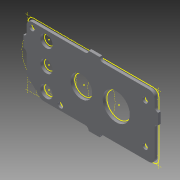
# Autodesk Inventor part: Granny Gearbox Output Plate Routing Template (border tabs)
Saved by Autodesk Inventor 2015 (Build 190159000, 159)
## iProperties
Created: 2016-02-25
Part Number: Granny Gearbox Output Plate Routing Template (border tabs)
Material: Generic
Document SubType Name: Modeling
Designer: sethbattis
Density: 1 g/cm^3
Appearance: Default
Author: sethbattis
Autodesk Inventor part; units mm, degrees
ref_plane "YZ Plane" through (0, 0, 0) normal (1, 0, 0) x (0, 1, 0)
ref_plane "XZ Plane" through (0, 0, 0) normal (0, 1, 0) x (-1, 0, 0)
ref_plane "XY Plane" through (0, 0, 0) normal (0, 0, 1) x (1, 0, 0)
derived "Granny Gearbox Output Plate.ipt"
sketch "New Mounting Holes" plane through (0, 0, 0) normal (0, 0, 1) x (1, 0, 0)
  circle A0 centre (74.3367, 23.3553) radius 3.175
  circle A1 centre (74.3367, -23.3553) radius 3.175
  circle A2 centre (-57.7242, 30.4609) radius 3.175
  circle A3 centre (-24.3812, -30.912) radius 3.175
  line L0 (-65.3633, -38.1) -> (-65.3633, 38.1) construction
  line L1 (87.0367, -38.1) -> (-65.3633, -38.1) construction
  line L2 (87.0367, 38.1) -> (87.0367, -38.1) construction
  line L3 (-65.3633, 38.1) -> (87.0367, 38.1) construction
  line L4 (-55.8383, 38.1) -> (-55.8383, -38.1) construction
  line L5 (-65.3633, 28.575) -> (87.0367, 28.575) construction
  line L6 (-65.3633, -28.575) -> (87.0367, -28.575) construction
  line L7 (77.5117, 38.1) -> (77.5117, -38.1) construction
  circle A4 centre (-40.7035, -0.0359) radius 31.75 construction
  circle A5 centre (40.6908, 0) radius 36.195 construction
  circle A6 centre (0, 0) radius 36.195 construction
  line L8 (-57.7242, 30.4609) -> (-55.8383, 30.4609) construction
  line L9 (-57.7242, 30.4609) -> (-57.7242, 28.575) construction
sketch "Labels" plane through (0, 0, 0) normal (0, 0, 1) x (1, 0, 0)
  circle A0 centre (-40.7035, -0.0359) radius 5.5626
  circle A1 centre (-40.7035, 25.3641) radius 5.5626
  circle A2 centre (-40.7035, -25.4359) radius 5.5626
  circle A3 centre (0, 0) radius 11.1125
  circle A4 centre (40.6908, 0) radius 14.2875
  line L0 (-5.8677, 26.2224) -> (48.5566, 26.2224) construction
  line L1 (48.5566, 26.2224) -> (48.5566, 22.1963) construction
  line L2 (48.5566, 22.1963) -> (-5.8677, 22.1963) construction
  line L3 (-5.8677, 22.1963) -> (-5.8677, 26.2224) construction
sketch "Exterior" plane through (0, 0, 0) normal (0, 0, 1) x (1, 0, 0)
  line L0 (-59.0133, 38.1) -> (80.6867, 38.1)
  line L1 (87.0367, 31.75) -> (87.0367, -31.75)
  line L2 (80.6867, -38.1) -> (-44.6678, -38.1)
  arc A0 (87.0367, 31.75) -> (80.6867, 38.1) centre (80.6867, 31.75) ccw
  arc A1 (80.6867, -38.1) -> (87.0367, -31.75) centre (80.6867, -31.75) ccw
  arc A2 (-59.0133, 38.1) -> (-65.3633, 31.75) centre (-59.0133, 31.75) ccw
  circle A3 centre (-40.7035, -0.0359) radius 31.75 construction
  line L3 (-65.3633, -17.4045) -> (-65.3633, 31.75)
  line L4 (-63.5034, -21.8946) -> (-49.1579, -36.2401)
  line L5 (-65.3633, -38.1) -> (-65.3633, 38.1) construction
  line L6 (87.0367, -38.1) -> (-65.3633, -38.1) construction
  arc A4 (-49.1579, -36.2401) -> (-44.6678, -38.1) centre (-44.6678, -31.75) ccw
  arc A5 (-65.3633, -17.4045) -> (-63.5034, -21.8946) centre (-59.0133, -17.4045) ccw
  point P0 (87.0367, 38.1)
  point P1 (-65.3633, -20.0348)
  point P2 (-47.2981, -38.1)
sketch "Sketch1" plane through (0, 0, 0) normal (0, 0, 1) x (1, 0, 0)
  circle A0 centre (-57.7242, 30.4609) radius 3.175 projected
  circle A1 centre (74.3367, 23.3553) radius 3.175 projected
  circle A2 centre (74.3367, -23.3553) radius 3.175 projected
  circle A3 centre (-24.3812, -30.912) radius 3.175 projected
  circle A4 centre (-40.7035, 25.3641) radius 7.0866
  circle A5 centre (-40.7035, -0.0359) radius 7.0866
  circle A6 centre (-40.7035, -25.4359) radius 7.0866
  circle A7 centre (0, 0) radius 12.6365
  circle A8 centre (40.6908, 0) radius 15.8115
  circle A9 centre (74.3367, 23.3553) radius 3.175
  circle A10 centre (74.3367, -23.3553) radius 3.175
  circle A11 centre (-24.3812, -30.912) radius 3.175
  circle A12 centre (-57.7242, 30.4609) radius 3.175
  circle A13 centre (-40.7035, -0.0359) radius 5.5626 projected
  circle A14 centre (-40.7035, -25.4359) radius 5.5626 projected
  circle A15 centre (-40.7035, 25.3641) radius 5.5626 projected
  circle A16 centre (0, 0) radius 11.1125 projected
  circle A17 centre (40.6908, 0) radius 14.2875 projected
  line L0 (-57.4893, 36.576) -> (4.5912, 36.576)
  line L1 (85.5127, 30.226) -> (85.5127, 22.2463)
  line L2 (79.1627, -36.576) -> (25.2287, -36.576)
  line L3 (-65.3633, 38.1) -> (87.0367, 38.1) construction
  line L4 (87.0367, 38.1) -> (87.0367, -38.1) construction
  line L5 (87.0367, -38.1) -> (-65.3633, -38.1) construction
  line L6 (-63.5034, -21.8946) -> (-49.1579, -36.2401) projected
  line L7 (-65.3633, -38.1) -> (-65.3633, 38.1) construction
  line L8 (-61.9794, -21.2634) -> (-48.5267, -34.7161)
  line L9 (-63.8393, -16.7732) -> (-63.8393, 1.6088)
  arc A18 (-57.4893, 36.576) -> (-63.8393, 30.226) centre (-57.4893, 30.226) ccw
  arc A19 (-63.8393, -16.7732) -> (-61.9794, -21.2634) centre (-57.4893, -16.7732) ccw
  arc A20 (-48.5267, -34.7161) -> (-44.0365, -36.576) centre (-44.0365, -30.226) ccw
  arc A21 (79.1627, -36.576) -> (85.5127, -30.226) centre (79.1627, -30.226) ccw
  arc A22 (85.5127, 30.226) -> (79.1627, 36.576) centre (79.1627, 30.226) ccw
  line L10 (21.2599, 40.5448) -> (21.2599, 40.5448)
  line L11 (21.2599, 40.5448) -> (8.5599, 40.5448)
  line L12 (8.5599, 40.5448) -> (8.5599, 40.5448)
  line L13 (21.2599, -40.5447) -> (21.2599, -40.5447)
  line L14 (21.2599, -40.5447) -> (8.5599, -40.5448)
  line L15 (8.5599, -40.5448) -> (8.5599, -40.5448)
  line L16 (25.2287, 36.576) -> (79.1627, 36.576)
  line L17 (4.5912, -36.576) -> (-44.0365, -36.576)
  arc A23 (4.5912, 36.576) -> (8.5599, 40.5448) centre (4.5912, 40.5448) ccw
  arc A24 (21.2599, 40.5448) -> (25.2287, 36.576) centre (25.2287, 40.5448) ccw
  arc A25 (8.5599, -40.5448) -> (4.5912, -36.576) centre (4.5912, -40.5448) ccw
  arc A26 (25.2287, -36.576) -> (21.2599, -40.5447) centre (25.2287, -40.5448) ccw
  line L18 (-67.808, 18.2775) -> (-67.808, 18.2775)
  line L19 (-67.808, 18.2775) -> (-67.808, 5.5775)
  line L20 (-67.808, 5.5775) -> (-67.808, 5.5775)
  line L21 (-63.8393, 22.2463) -> (-63.8393, 30.226)
  line L22 (89.4815, 18.2775) -> (89.4815, 18.2775)
  line L23 (89.4815, 18.2775) -> (89.4815, 5.5775)
  line L24 (89.4815, 5.5775) -> (89.4815, 5.5775)
  line L25 (85.5127, 1.6088) -> (85.5127, -30.226)
  arc A27 (-67.808, 18.2775) -> (-63.8393, 22.2463) centre (-67.808, 22.2463) ccw
  arc A28 (-63.8393, 1.6088) -> (-67.808, 5.5775) centre (-67.808, 1.6088) ccw
  arc A29 (85.5127, 22.2463) -> (89.4815, 18.2775) centre (89.4815, 22.2463) ccw
  arc A30 (89.4815, 5.5775) -> (85.5127, 1.6088) centre (89.4815, 1.6088) ccw
  point P0 (21.2599, 36.576)
  point P1 (21.2599, -36.576)
  point P2 (-63.8393, 18.2775)
  point P3 (85.5127, 5.5775)
  dimension "d15" = 1.524
  dimension "d18" = 1.524
  dimension "d19" = 1.524
  dimension "d21" = 1.524
  dimension "d22" = 6.35
  dimension "d23" = 28.575
  dimension "d24" = 31.623
  dimension "d25" = 22.225
  dimension "d26" = 25.273
  dimension "d27" = 11.1252
  dimension "d28" = 14.1732
  dimension "d31" = 12.7
  dimension "d32" = 3.9688
  dimension "d33" = 12.7
  dimension "d34" = 3.9688
  dimension "d35" = 3.9688
  dimension "d36" = 3.9688
  dimension "d37" = 12.7
  dimension "d38" = 3.9688
  dimension "d39" = 3.9688
  constraints: 42 end point, 34 tangent, 26 point on circle, 22 centre point, 16 equal radius, 13 parallel, 9 coincident, 8 point on line, 6 perpendicular, 5 concentric, 4 horizontal, 1 collinear
  measures "d15" distance between parallel lines of L0 L3
  measures "d18" distance between parallel lines of L1 L4
  measures "d19" distance between parallel lines of L5 L2
  measures "d21" distance between parallel lines of L8 L6
  measures "d22" radius of A18
  measures "d23" diameter of A17
  measures "d24" diameter of A8
  measures "d25" diameter of A16
  measures "d26" diameter of A7
  measures "d27" diameter of A15
  measures "d28" diameter of A4
  measures "d31" distance of L11.end L10.end
  measures "d32" distance of L10.end point (21.26, 36.576)
  measures "d33" distance of L13.end L14.end
  measures "d34" distance of point (21.26, -36.576) L13.end
  measures "d35" radius of A23
  measures "d36" distance of point (-63.839, 18.278) L18.end
  measures "d37" distance of L18.end L19.end
  measures "d38" distance of L23.end point (85.513, 5.578)
  measures "d39" radius of A27
extrude "Extrusion1" add sketch "Sketch1" along normal blind 3.175 contours L0 A23 L11 A24 L16 A22 L1 A29 L23 A30 L25 A21 L2 A26 L14 A25 L17 A20 L8 A19 L9 A28 L19 A27 L21 A18
equation "\"d18\" = d15"
equation "\"d19\" = d15"
equation "\"d21\" = d15"
equation "\"d24\" = d23 + 2 * d15"
equation "\"d26\" = d25 + 2 * d15"
equation "\"d28\" = d27 + 2 * d15"
body "Solid2"
